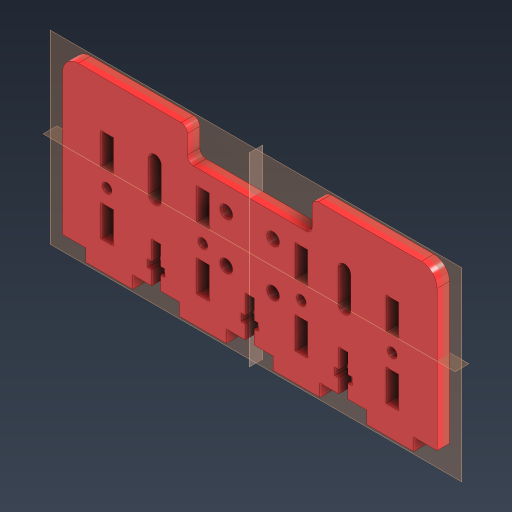
# Autodesk Inventor part: Выступ_под_крепление_маркера
Saved by Autodesk Inventor 2023.2 (Build 272271030, 271C)
## iProperties
Created: 2025-12-29
Part Number: Выступ_под_крепление_маркера
Material: Типовые
Document SubType Name: Modeling
Designer: Олег Коноваленко
Density: 1 g/cm^3
Appearance: Светло-красный
Author: Олег Коноваленко
Autodesk Inventor part; units mm, degrees
sketch "Эскиз1" plane through (0, 0, 0) normal (0, 0, 1) x (1, 0, 0)
  line L0 (-60, 25) -> (60, 25)
  line L1 (60, 25) -> (60, -25)
  line L2 (60, -25) -> (-60, -25)
  line L3 (-60, -25) -> (-60, 25)
  line L4 (-60, 25) -> (60, -25) construction
  line L5 (60, 25) -> (-60, -25) construction
  point P0 (0, 0)
  dimension "d0" = 120
  dimension "d1" = 50
  constraints: 12 end point, 2 midpoint, 2 parallel, 1 horizontal, 1 perpendicular
  measures "d0" distance of L0.start L0.end
  measures "d1" distance of L2.end L0.start
extrude "Выдавливание1" add sketch "Эскиз1" along normal mid plane 4
sketch "Эскиз2" plane through (0, 0, 2) normal (0, 0, 1) x (1, 0, 0)
  line L0 (-60, -25) -> (60, -25) projected
  line L1 (-52.5, -25) -> (-37.5, -25)
  line L2 (-37.5, -25) -> (-37.5, -29)
  line L3 (-37.5, -29) -> (-52.5, -29)
  line L4 (-52.5, -29) -> (-52.5, -25)
  line L5 (-22.5, -25) -> (-7.5, -25)
  line L6 (-7.5, -25) -> (-7.5, -29)
  line L7 (-7.5, -29) -> (-22.5, -29)
  line L8 (-22.5, -29) -> (-22.5, -25)
  line L9 (7.5, -25) -> (22.5, -25)
  line L10 (22.5, -25) -> (22.5, -29)
  line L11 (22.5, -29) -> (7.5, -29)
  line L12 (7.5, -29) -> (7.5, -25)
  line L13 (37.5, -25) -> (52.5, -25)
  line L14 (52.5, -25) -> (52.5, -29)
  line L15 (52.5, -29) -> (37.5, -29)
  line L16 (37.5, -29) -> (37.5, -25)
  point P0 (0, 0)
  dimension "d4" = 4
  dimension "d5" = 15
  dimension "d6" = 7.5
  dimension "d9" = 30
  constraints: 32 end point, 2 horizontal, 2 parallel, 1 perpendicular, 1 point on line, 24 other
  measures "d4" distance of L3.end L1.start
  measures "d5" distance of L2.end L3.end
  measures "d6" distance from line of L0.start L4
  measures "d9" distance of L1.start L5.start
extrude "Выдавливание2" add sketch "Эскиз2" against normal up to surface (4 mm away)
sketch "Эскиз3" plane through (0, 0, 2) normal (0, 0, 1) x (1, 0, 0)
  line L0 (-22.5, -25) -> (-37.5, -25) projected
  line L1 (-28.55, -25) -> (-31.45, -25)
  line L2 (-31.45, -25) -> (-31.45, -12)
  line L3 (-31.45, -12) -> (-28.55, -12)
  line L4 (-28.55, -12) -> (-28.55, -25)
  line L5 (7.5, -25) -> (-7.5, -25) projected
  line L6 (1.45, -25) -> (-1.45, -25)
  line L7 (-1.45, -25) -> (-1.45, -12)
  line L8 (-1.45, -12) -> (1.45, -12)
  line L9 (1.45, -12) -> (1.45, -25)
  line L10 (31.45, -25) -> (28.55, -25)
  line L11 (28.55, -25) -> (28.55, -12)
  line L12 (28.55, -12) -> (31.45, -12)
  line L13 (31.45, -12) -> (31.45, -25)
  line L14 (22.5, -25) -> (37.5, -25) projected
  line L15 (-32.8, -18.2) -> (-27.2, -18.2)
  line L16 (-27.2, -18.2) -> (-27.2, -20.5)
  line L17 (-27.2, -20.5) -> (-32.8, -20.5)
  line L18 (-32.8, -20.5) -> (-32.8, -18.2)
  line L19 (-2.8, -18.2) -> (2.8, -18.2)
  line L20 (2.8, -18.2) -> (2.8, -20.5)
  line L21 (2.8, -20.5) -> (-2.8, -20.5)
  line L22 (-2.8, -20.5) -> (-2.8, -18.2)
  line L23 (27.2, -18.2) -> (32.8, -18.2)
  line L24 (32.8, -18.2) -> (32.8, -20.5)
  line L25 (32.8, -20.5) -> (27.2, -20.5)
  line L26 (27.2, -20.5) -> (27.2, -18.2)
  line L27 (30, -12) -> (30, -25) construction
  line L28 (-30, -12) -> (-30, -25)
  line L29 (0, 35.8) -> (0, -39.8) projected
  point P0 (0, 0)
  point P1 (0, -25)
  point P2 (-30, -18.2)
  point P3 (0, -18.2)
  point P4 (30, -18.2)
  point P5 (28.55, -20.5)
  point P6 (31.45, -20.5)
  point P7 (31.45, -18.2)
  point P8 (28.55, -18.2)
  point P9 (1.45, -18.2)
  point P10 (-1.45, -18.2)
  point P11 (-1.45, -20.5)
  point P12 (1.45, -20.5)
  point P13 (-31.45, -20.5)
  point P14 (-28.55, -20.5)
  point P15 (-28.55, -18.2)
  point P16 (-31.45, -18.2)
  dimension "d16" = 2.9
  dimension "d17" = 13
  dimension "d18" = 5.6
  dimension "d19" = 2.3
  dimension "d20" = 4.5
  dimension "d21" = 4.5
  dimension "d22" = 4.5
  constraints: 52 end point, 13 parallel, 11 midpoint, 8 equal length, 6 horizontal, 6 perpendicular, 5 point on line, 1 vertical
  measures "d16" distance of L11.end L12.end
  measures "d17" distance of L12.end L10.start
  measures "d18" distance of L24.end L25.end
  measures "d19" distance of L23.end L24.end
  measures "d20" distance between parallel lines of L14 L25
  measures "d21" distance between parallel lines of L5 L21
  measures "d22" distance between parallel lines of L0 L17
extrude "Выдавливание3" cut sketch "Эскиз3" against normal up to next
sketch "Эскиз4" plane through (0, 0, 2) normal (0, 0, 1) x (1, 0, 0)
  line L0 (-43.7, 0) -> (-47.7, 0) projected
  line L1 (-43.7, 10) -> (-43.7, 0) projected
  line L2 (-47.7, 10) -> (-43.7, 10) projected
  line L3 (-47.7, 0) -> (-47.7, 10) projected
  line L4 (-47.7, -20) -> (-43.7, -20) projected
  line L5 (-43.7, -10) -> (-43.7, -20) projected
  line L6 (-47.7, -10) -> (-43.7, -10) projected
  line L7 (-47.7, -20) -> (-47.7, -10) projected
  line L8 (47.7, 0) -> (43.7, 0) projected
  line L9 (47.7, 10) -> (47.7, 0) projected
  line L10 (43.7, 10) -> (47.7, 10) projected
  line L11 (43.7, 0) -> (43.7, 10) projected
  line L12 (43.7, -20) -> (47.7, -20) projected
  line L13 (47.7, -10) -> (47.7, -20) projected
  line L14 (43.7, -10) -> (47.7, -10) projected
  line L15 (43.7, -20) -> (43.7, -10) projected
  line L16 (-13, 0) -> (-17, 0) projected
  line L17 (-13, 10) -> (-13, 0) projected
  line L18 (-17, 10) -> (-13, 10) projected
  line L19 (-17, 0) -> (-17, 10) projected
  line L20 (-17, -20) -> (-13, -20) projected
  line L21 (-13, -10) -> (-13, -20) projected
  line L22 (-17, -10) -> (-13, -10) projected
  line L23 (-17, -20) -> (-17, -10) projected
  line L24 (14.55, -20) -> (18.55, -20) projected
  line L25 (18.55, -10) -> (18.55, -20) projected
  line L26 (14.55, -10) -> (18.55, -10) projected
  line L27 (14.55, -20) -> (14.55, -10) projected
  line L28 (18.55, 0) -> (14.55, 0) projected
  line L29 (18.55, 10) -> (18.55, 0) projected
  line L30 (14.55, 10) -> (18.55, 10) projected
  line L31 (14.55, 0) -> (14.55, 10) projected
extrude "Выдавливание4" cut sketch "Эскиз4" against normal up to next
sketch "Эскиз5" plane through (0, 0, 2) normal (0, 0, 1) x (1, 0, 0)
  line L0 (-84, 0) -> (84, 0) construction
  line L1 (-45.7, 35.8) -> (-45.7, -39.8) construction
  line L2 (45.7, 35.8) -> (45.7, -39.8) construction
  line L3 (-43.7, 0) -> (-47.7, 0) projected
  line L4 (-47.7, -10) -> (-43.7, -10) projected
  line L5 (43.7, -10) -> (47.7, -10) projected
  line L6 (47.7, 0) -> (43.7, 0) projected
  line L7 (-45.7, 0) -> (-45.7, -10) construction
  line L8 (-43.7, -10) -> (-47.7, -10) projected
  line L9 (45.7, 0) -> (45.7, -10) construction
  circle A0 centre (-45.7, -5) radius 1.5
  circle A1 centre (45.7, -5) radius 1.5
  line L10 (-17, 0) -> (-13, 0) projected
  line L11 (-15, 0) -> (-15, -10) construction
  line L12 (-13, -10) -> (-17, -10) projected
  circle A2 centre (-15, -5) radius 1.5
  line L13 (14.55, 0) -> (18.55, 0) projected
  line L14 (16.55, 0) -> (16.55, -10) construction
  line L15 (18.55, -10) -> (14.55, -10) projected
  circle A3 centre (16.55, -5) radius 1.5
  dimension "d30" = 3
  constraints: 12 end point, 12 midpoint, 4 centre point, 3 equal radius, 2 vertical, 5 other
  measures "d30" diameter of A0
extrude "Выдавливание5" cut sketch "Эскиз5" against normal up to next
sketch "Эскиз7" plane through (0, 0, -2) normal (0, 0, -1) x (-1, 0, 0)
  line L0 (60, 25) -> (-60, 25) projected
  arc A0 (-17.8, 23.5) -> (-16.8, 22.5) centre (-16.8, 23.5) ccw projected
  line L1 (-16.8, 22.5) -> (-15.6382, 22.5) projected
  arc A1 (-14.8497, 22.115) -> (-15.6382, 22.5) centre (-15.6382, 21.5) ccw
  line L2 (-14.8497, 22.115) -> (-11.5503, 17.885) projected
  arc A2 (-11.5503, 17.885) -> (-10.7618, 17.5) centre (-10.7618, 18.5) ccw projected
  line L3 (-10.7618, 17.5) -> (10.7618, 17.5) projected
  arc A3 (10.7618, 17.5) -> (11.5503, 17.885) centre (10.7618, 18.5) ccw projected
  line L4 (11.5503, 17.885) -> (14.8497, 22.115) projected
  arc A4 (15.6382, 22.5) -> (14.8497, 22.115) centre (15.6382, 21.5) ccw projected
  line L5 (15.6382, 22.5) -> (16.8, 22.5) projected
  arc A5 (16.8, 22.5) -> (17.8, 23.5) centre (16.8, 23.5) ccw projected
  line L6 (17.8, 23.5) -> (17.8, 34.5) projected
  line L7 (-20, 15) -> (20, 15)
  line L8 (20, 15) -> (20, 25)
  line L9 (20, 25) -> (-20, 25)
  line L10 (-20, 25) -> (-20, 15)
  line L11 (-20, 15) -> (20, 25) construction
  line L12 (20, 15) -> (-20, 25) construction
  line L13 (0, -41.7) -> (0, 47.2) construction
  point P0 (0, 0)
  point P1 (0, 20)
  point P2 (-20, 25)
  dimension "d37" = 40
  dimension "d38" = 10
  constraints: 12 end point, 2 midpoint, 2 parallel, 2 point on circle, 2 point on line, 1 centre point, 1 horizontal, 1 perpendicular
  measures "d37" distance of L7.start L7.end
  measures "d38" distance of L9.end L7.start
extrude "Выдавливание7" cut sketch "Эскиз7" against normal up to next
fillet "Сопряжение1" radius 2 4 edges at (20, 15, 0) (20, 25, 0) (-20, 25, 0) (-20, 15, 0)
sketch "Эскиз8" plane through (0, 0, -2) normal (0, 0, -1) x (-1, 0, 0)
  circle A0 centre (-7.5, 7.5) radius 2
  circle A1 centre (7.5, 7.5) radius 2
  circle A2 centre (-7.5, -7.5) radius 2
  circle A3 centre (7.5, -7.5) radius 2
  line L0 (-7.5, 7.5) -> (-7.5, -7.5) construction
  line L1 (-7.5, -7.5) -> (7.5, -7.5) construction
  line L2 (7.5, -7.5) -> (7.5, 7.5) construction
  line L3 (7.5, 7.5) -> (-7.5, 7.5) construction
  line L4 (-7.5, 7.5) -> (7.5, -7.5) construction
  line L5 (7.5, 7.5) -> (-7.5, -7.5) construction
  point P0 (0, 0)
  point P1 (0, 0)
  dimension "d42" = 4
  dimension "d43" = 15
  constraints: 12 end point, 4 centre point, 4 perpendicular, 3 equal radius, 1 coincident, 1 horizontal, 1 midpoint
  measures "d42" diameter of A0
  measures "d43" distance of L2.end L0.start
extrude "Выдавливание8" cut sketch "Эскиз8" against normal up to next
fillet "Сопряжение2" radius 5 2 edges at (60, 25, 0) (-60, 25, 0)
sketch "Эскиз9" plane through (0, 0, 2) normal (0, 0, 1) x (1, 0, 0)
  line L0 (-30.35, 0) -> (-30.35, 10) construction
  line L1 (-28.35, 0) -> (-28.35, 10)
  line L2 (-32.35, 10) -> (-32.35, 0)
  arc A0 (-32.35, 0) -> (-28.35, 0) centre (-30.35, 0) ccw
  arc A1 (-28.35, 10) -> (-32.35, 10) centre (-30.35, 10) ccw
  line L3 (-43.7, 10) -> (-43.7, 0) projected
  line L4 (-17, 0) -> (-17, 10) projected
  line L5 (-84, 0) -> (84, 0) construction
  point P0 (0, 0)
  point P1 (-30.35, 5)
  dimension "d47" = 10
  dimension "d48" = 2
  dimension "d50" = 13.35
  dimension "d51" = 5
  constraints: 8 end point, 4 point on circle, 4 tangent, 2 centre point, 1 midpoint, 1 parallel, 1 vertical
  measures "d47" distance of L0.start L0.end
  measures "d48" distance between parallel lines of L2 L0
  measures "d50" distance from line of point (-30.35, 5) L4
  measures "d51" distance from line of L5 point (-30.35, 5)
extrude "Выдавливание9" cut sketch "Эскиз9" against normal up to next
mirror "Зеркальное отражение1" about plane through (0, 0, 0) normal (1, 0, 0) of "Выдавливание9"
